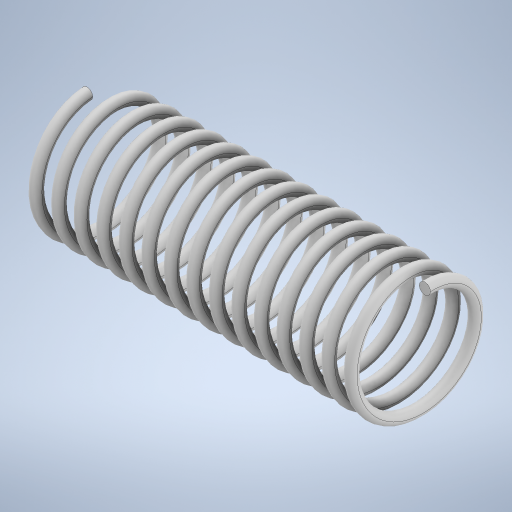
# Autodesk Inventor part: Hudson 1-61
Saved by Autodesk Inventor 2024.2 (Build 282272000, 272)
## iProperties
Created: 2024-10-07
Part Number: Hudson 1-61
Material: Genérico
Document SubType Name: Modeling
Designer: Monica Mora
Density: 1 g/cm^3
Appearance: Valor por defecto
Author: Monica Mora
Autodesk Inventor part; units mm, degrees
ref_plane "YZ Plane" through (0, 0, 0) normal (1, 0, 0) x (0, 1, 0)
ref_plane "XZ Plane" through (0, 0, 0) normal (0, 1, 0) x (-1, 0, 0)
ref_plane "XY Plane" through (0, 0, 0) normal (0, 0, 1) x (1, 0, 0)
sketch "Boceto1" plane through (0, 0, 0) normal (0, 0, 1) x (1, 0, 0)
  line L0 (0, 0) -> (-6.3438, 0)
  circle A0 centre (0, 2.5) radius 0.25
  dimension "d0" = 5
  dimension "d1" = 0.5
  constraints: 2 end point, 1 centre point, 1 horizontal
  measures "d0" diameter of A0.centre L0
  measures "d1" diameter of A0
coil "Bobina1" sketch "Boceto1" operation add axis through (0, 0, 0) along (-1, 0, 0) pitch 1 turns 15 hand right
